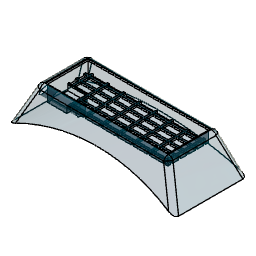
Aquazepp_LEDDisplay v6 (Autodesk Fusion 360 design; units mm, degrees)
Autodesk Fusion 360 part; units mm, degrees
note: some values were not read from the file. Set by a fixed rule: which sketch regions a step uses.
sketch "Skizze1" plane through (0, 0, 0) normal (0, 0, 1) x (1, 0, 0)
  line L0 (-36, 12.1) -> (36, 12.1)
  line L1 (36, 12.1) -> (36, -12.1)
  line L2 (36, -12.1) -> (-36, -12.1)
  line L3 (-36, -12.1) -> (-36, 12.1)
  line L4 (0, 0) -> (0, 52.2581) construction
  line L5 (0, 0) -> (51.3724, 0) construction
  line L6 (39, -15.1) -> (-39, -15.1)
  line L7 (-39, -15.1) -> (-39, 15.1)
  line L8 (-39, 15.1) -> (39, 15.1)
  line L9 (39, 15.1) -> (39, -15.1)
  dimension "d1" = 72
  dimension "d2" = 24.2
  dimension "d3" = -3
  constraint horizontal L0
  constraint vertical L1
  constraint horizontal L2
  constraint vertical L3
  constraint coincident L4.start L5.start
  constraint perpendicular L0 L4
  constraint perpendicular L1 L5
  constraint symmetric L1 L3 L4
  constraint symmetric L0 L2 L5
  measures "d1" distance of L0.start L0.end
  measures "d2" distance of L0.start L2.end
extrude "Extrusion1" add sketch "Skizze1" along normal blind 12
extrude "Extrusion5" add sketch "Skizze1" along normal blind 5 contours L0 L1 L2 L3
extrude "Extrusion6" add sketch "Skizze1" against normal blind 13 contours L0 L1 L2 L3 | L6 L7 L8 L9
sketch "Skizze4" plane through (-39, 0, 0) normal (-1, 0, 0) x (0, -1, 0)
  line L0 (15.1, -13) -> (15.1, 12)
  line L1 (15.1, 12) -> (-15.1, 12)
  line L2 (-15.1, 12) -> (-15.1, -13)
  line L3 (-15.1, -13) -> (15.1, -13)
  line L4 (12.6192, 12) -> (0, 0) construction
  line L5 (0, 12) -> (12.3356, 0.4524) construction
  line L6 (6.3096, 6) -> (6.3096, -2.5026) construction
  circle A0 centre (6.3096, 1.7487) radius 2.85
  dimension "d17" = 5.7
  constraint coincident L1 L4.start
  constraint coincident L4.end origin
  constraint midpoint L1 L5.start
  constraint midpoint L4 L6.start
  constraint vertical L6
  constraint midpoint L6 A0.centre
  measures "d17" diameter of A0
sketch "Skizze5" plane through (0, 0, 5) normal (0, 0, 1) x (-1, 0, 0)
  line L0 (36, 12.1) -> (-36, 12.1)
  line L1 (-36, 12.1) -> (-36, -12.1)
  line L2 (-36, -12.1) -> (36, -12.1)
  line L3 (36, -12.1) -> (36, 12.1)
  line L4 (-36, 12.1) -> (36, 12.1)
  line L5 (36, 12.1) -> (36, -12.1)
  line L6 (-36, 12.1) -> (36, 12.1)
  line L7 (36, 12.1) -> (36, -12.1)
  line L8 (36, 0) -> (24.5, 0)
  line L9 (24.5, 0) -> (24.5, 12.1)
  dimension "d18" = 11.5
  dimension "d68" = 12.1
  constraint midpoint L5 L8.start
  constraint perpendicular L7 L8
  constraint coincident L6 L9.end
  constraint perpendicular L6 L9
  measures "d18" distance of L8.start L8.end
  measures "d68" distance of L8.end L9.end
extrude "Extrusion8" cut sketch "Skizze5" against normal blind 3 contours L0 L3 L4 L5 L6 L7 L8 L9
sketch "Skizze6" plane through (0, -15.1, 0) normal (0, -1, 0) x (1, 0, 0)
  line L0 (39, -13) -> (39, 12)
  line L1 (39, 12) -> (-39, 12)
  line L2 (-39, 12) -> (-39, -13)
  line L3 (-39, -13) -> (39, -13)
  circle A0 centre (0, -115) radius 115.5
  line L4 (-36, 5) -> (36, 5)
  line L5 (-39, 12) -> (-49.5461, -10.6667)
  line L6 (0, 0) -> (0, 57.4793) construction
  line L7 (39, 12) -> (49.5461, -10.6667)
  dimension "d23" = 231
  dimension "d24" = 120
  dimension "d31" = 25
  constraint coincident L1.end L2.start
  constraint coincident A0 L5.end
  constraint coincident L6.start origin
  constraint perpendicular L4 L6
  constraint symmetric L1.end L6 L0.end
  constraint symmetric L5.end L6 L7.end
  measures "d23" diameter of A0
  measures "d24" distance of A0.centre L4
  measures "d31" distance of L1.end L5.end
sketch "Skizze7" plane through (-39, 0, -1.5) normal (-1, 0, 0) x (0, -1, 0)
  line L0 (15.1, 13.5) -> (-15.1, 13.5)
  line L1 (-15.1, 13.5) -> (-15.1, -11.5)
  line L2 (15.1, 13.5) -> (15.1, -9.1667)
  line L3 (-15.1, 13.5) -> (-22.3824, -10.4158)
  line L4 (-22.3824, -10.4158) -> (-15.1, -11.5)
  line L5 (0, 6.5) -> (0, 3.5)
  line L6 (15.1, 13.5) -> (22.3824, -10.4158)
  line L7 (22.3824, -10.4158) -> (15.1, -11.5)
  line L8 (15.1, -229) -> (15.1, 2)
  line L9 (15.1, 1.5) -> (15.1, 58.9793)
  line L10 (15.1, 13.5) -> (24.8067, 41.0778)
  line L11 (24.8067, 41.0778) -> (71.9975, -14.9794)
  line L12 (71.9975, -14.9794) -> (37.33, -35.3345)
  line L13 (37.33, -35.3345) -> (22.3824, -10.4158)
  line L14 (-15.1, 13.5) -> (-24.8067, 41.0778)
  line L15 (-24.8067, 41.0778) -> (-71.9975, -14.9794)
  line L16 (-71.9975, -14.9794) -> (-37.33, -35.3345)
  line L17 (-37.33, -35.3345) -> (-22.3824, -10.4158)
  dimension "d32" = 25
  constraint coincident L0.end L1.start
  constraint coincident L1.end L4.end
  constraint symmetric L0.end L5 L0.start
  constraint symmetric L3.end L5 L6.end
  constraint symmetric L1.end L5 L7.end
  constraint coincident L0.start L2.start
  constraint symmetric L5 L6.end L3.end
  constraint symmetric L5 L0.start L0.end
  constraint symmetric L5 L10.end L14.end
  constraint symmetric L5 L11.end L15.end
  constraint symmetric L5 L12.end L16.end
  measures "d32" distance of L0.end L3.end
extrude "Extrusion10" add sketch "Skizze7" against normal blind 78 contours L1 L3 L4 | L2 L6 L7 L8 L9
extrude "Extrusion11" add sketch "Skizze6" against normal blind 40 contours L0 A0 L7 | L2 A0 L5
extrude "Extrusion12" add 2 faces at (40.1876, -15.1, -0.6374) (-40.1876, -15.1, -0.6374) along direction (0, -1, 0) blind 10
extrude "Extrusion9" cut sketch "Skizze6" along normal mid plane 104 contours L0 L2 L3 A0 | L0 L2 L3 A0
extrude "Extrusion13" cut sketch "Skizze7" along normal mid plane 212 contours L3 L14 L15 L16 L17 | L6 L10 L11 L12 L13
extrude "Extrusion7" cut sketch "Skizze4" along normal mid plane 34 contours A0
fillet "Abrundung1" radius 3 8 edges at (0, -15.1, 12) (-39, 0, 12) (0, 15.1, 12) (39, 0, 12) (44.273, -18.551, 0.6666) (44.273, 18.551, 0.6666) (-44.273, 18.551, 0.6666) (-44.273, -18.551, 0.6666)
sketch "Skizze8" plane through (0, 0, 5) normal (0, 0, 1) x (1, 0, 0)
  line L0 (-36, -12.1) -> (-36, 12.1)
  line L1 (-36, 12.1) -> (36, 12.1)
  line L2 (-36, 0) -> (-24.5, 0)
  line L3 (-24.5, 0) -> (-24.5, -12.1)
  line L4 (36, -12.1) -> (-36, -12.1)
  line L5 (36, 12.1) -> (36, -12.1)
  line L6 (34.2972, 12.1) -> (34.2972, -12.1)
  line L7 (33.0972, 12.1) -> (33.0972, -12.1)
  line L8 (-36, 10.5188) -> (36, 10.5188)
  line L9 (36, 9.3188) -> (-36, 9.3188)
  line L10 (23.5258, 12.1) -> (23.5258, -12.1)
  line L11 (24.7258, 12.1) -> (24.7258, -12.1)
  line L12 (13.9544, 12.1) -> (13.9544, -12.1)
  line L13 (15.1544, 12.1) -> (15.1544, -12.1)
  line L14 (4.3829, 12.1) -> (4.3829, -12.1)
  line L15 (5.5829, 12.1) -> (5.5829, -12.1)
  line L16 (-5.1885, 12.1) -> (-5.1885, -12.1)
  line L17 (-3.9885, 12.1) -> (-3.9885, -12.1)
  line L18 (-14.7599, 12.1) -> (-14.7599, -12.1)
  line L19 (-13.5599, 12.1) -> (-13.5599, -12.1)
  line L20 (-24.3313, 12.1) -> (-24.3313, -12.1)
  line L21 (-23.1313, 12.1) -> (-23.1313, -12.1)
  line L22 (-33.9028, 12.1) -> (-33.9028, -12.1)
  line L23 (-32.7028, 12.1) -> (-32.7028, -12.1)
  line L24 (-36, 5.5188) -> (36, 5.5188)
  line L25 (36, 4.3188) -> (-36, 4.3188)
  line L26 (-36, 0.5188) -> (36, 0.5188)
  line L27 (36, -0.6812) -> (-36, -0.6812)
  line L28 (-36, -4.4812) -> (36, -4.4812)
  line L29 (36, -5.6812) -> (-36, -5.6812)
  line L30 (-36, -9.4812) -> (36, -9.4812)
  line L31 (36, -10.6812) -> (-36, -10.6812)
  dimension "d55" = 1.2
  dimension "d56" = 1.2
  dimension "d59" = -67
  dimension "d60" = 0
  dimension "d63" = 0
  dimension "d64" = -20
  constraint coincident L1 L6.start
  constraint coincident L4 L6.end
  constraint perpendicular L4 L6
  constraint coincident L1 L7.start
  constraint coincident L4 L7.end
  constraint perpendicular L1 L7
  constraint coincident L0 L8.start
  constraint coincident L5 L8.end
  constraint perpendicular L5 L8
  constraint coincident L5 L9.start
  constraint coincident L0 L9.end
  constraint perpendicular L0 L9
  measures "d55" distance of L8 L9
  measures "d56" distance of L6 L7
extrude "Extrusion15" add sketch "Skizze8" along normal blind 1 draft 1 contours L3 L20 L30 L31 | L4 L20 L21 L31 | L20 L21 L30 L31 | L0 L2 L22 L26 | L3 L20 L28 L29 | L20 L21 L29 L30 | L18 L21 L30 L31 | L4 L18 L19 L31 | L2 L22 L23 L26 | L20 L21 L28 L29 | L18 L19 L30 L31 | L0 L22 L24 L25 | L22 L23 L25 L26 | L2 L3 L20 L23 L26 L27 | L20 L21 L27 L28 | L18 L21 L28 L29 | L18 L19 L29 L30 | L16 L19 L30 L31 | L4 L16 L17 L31 | L22 L23 L24 L25 | L20 L21 L26 L27 | L18 L19 L28 L29 | L16 L17 L30 L31 | L0 L8 L9 L22 | L9 L22 L23 L24 | L20 L23 L24 L25 | L20 L21 L25 L26 | L18 L21 L26 L27 | L18 L19 L27 L28 | L16 L19 L28 L29 | L16 L17 L29 L30 | L14 L17 L30 L31 | L4 L14 L15 L31 | L8 L9 L22 L23 | L20 L21 L24 L25 | L18 L19 L26 L27 | L16 L17 L28 L29 | L14 L15 L30 L31 | L1 L8 L22 L23 | L8 L9 L20 L23 | L9 L20 L21 L24 | L18 L21 L24 L25 | L18 L19 L25 L26 | L16 L19 L26 L27 | L16 L17 L27 L28 | L14 L17 L28 L29 | L14 L15 L29 L30 | L12 L15 L30 L31 | L4 L12 L13 L31 | L8 L9 L20 L21 | L18 L19 L24 L25 | L16 L17 L26 L27 | L14 L15 L28 L29 | L12 L13 L30 L31 | L1 L8 L20 L21 | L8 L9 L18 L21 | L9 L18 L19 L24 | L16 L19 L24 L25 | L16 L17 L25 L26 | L14 L17 L26 L27 | L14 L15 L27 L28 | L12 L15 L28 L29 | L12 L13 L29 L30 | L10 L13 L30 L31 | L4 L10 L11 L31 | L8 L9 L18 L19 | L16 L17 L24 L25 | L14 L15 L26 L27 | L12 L13 L28 L29 | L10 L11 L30 L31 | L1 L8 L18 L19 | L8 L9 L16 L19 | L9 L16 L17 L24 | L14 L17 L24 L25 | L14 L15 L25 L26 | L12 L15 L26 L27 | L12 L13 L27 L28 | L10 L13 L28 L29 | L10 L11 L29 L30 | L7 L11 L30 L31 | L4 L6 L7 L31 | L8 L9 L16 L17 | L14 L15 L24 L25 | L12 L13 L26 L27 | L10 L11 L28 L29 | L6 L7 L30 L31 | L1 L8 L16 L17 | L8 L9 L14 L17 | L9 L14 L15 L24 | L12 L15 L24 L25 | L12 L13 L25 L26 | L10 L13 L26 L27 | L10 L11 L27 L28 | L7 L11 L28 L29 | L6 L7 L29 L30 | L5 L6 L30 L31 | L8 L9 L14 L15 | L12 L13 L24 L25 | L10 L11 L26 L27 | L6 L7 L28 L29 | L1 L8 L14 L15 | L8 L9 L12 L15 | L9 L12 L13 L24 | L10 L13 L24 L25 | L10 L11 L25 L26 | L7 L11 L26 L27 | L6 L7 L27 L28 | L5 L6 L28 L29 | L8 L9 L12 L13 | L10 L11 L24 L25 | L6 L7 L26 L27 | L1 L8 L12 L13 | L8 L9 L10 L13 | L9 L10 L11 L24 | L7 L11 L24 L25 | L6 L7 L25 L26 | L5 L6 L26 L27 | L8 L9 L10 L11 | L6 L7 L24 L25 | L1 L8 L10 L11 | L7 L8 L9 L11 | L6 L7 L9 L24 | L5 L6 L24 L25 | L6 L7 L8 L9 | L1 L6 L7 L8 | L5 L6 L8 L9
chamfer "Fase1" distance 0.5 angle 45 4 edges at (0, 12.1, 12) (-36, 0, 12) (0, -12.1, 12) (36, 0, 12)
equation "d2 = ( 12.1 * 2 ) * 1 mm"
equation "d33 = -72 mm - 6 mm"
equation "d56 = d55"
named bodies: "LEDDisplay"
